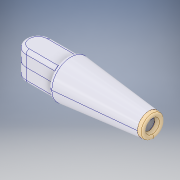
# Autodesk Inventor part: SimplifiedFoot040x
Saved by Autodesk Inventor 2018 (Build 220112000, 112)
## iProperties
Part Number: SimplifiedFoot040x
Material: PVC, hart
Document SubType Name: Modeling
Designer: Jochen Alt
Mass: 40.2314 g
Surface Area: 453.473 cm^2
Volume: 40.2314 cm^3
Density: 1.29 g/cm^3
Appearance: Glatt - waldgrün
Author: Jochen Alt
Autodesk Inventor part; units mm, degrees
(part 1 of 2)
ref_plane "YZ Plane" through (0, 0, 0) normal (1, 0, 0) x (0, 1, 0)
ref_plane "XZ Plane" through (0, 0, 0) normal (0, 1, 0) x (-1, 0, 0)
ref_plane "XY Plane" through (0, 0, 0) normal (0, 0, 1) x (1, 0, 0)
sketch "Skizze Servo Projektion" plane through (0, 0, 0) normal (0, 0, 1) x (1, 0, 0)
  circle A0 centre (6.3, 9) radius 0.85 construction
  circle A1 centre (6.3, -9) radius 0.85 construction
  circle A2 centre (-32.7, -9) radius 0.85 construction
  circle A3 centre (-32.7, 9) radius 0.85 construction
  circle A4 centre (-26.0282, 0) radius 9.5 construction
  line L0 (0.03, 10) -> (0.03, 11.5) construction
  arc A5 (0.03, 10) -> (1.9, 8.13) centre (1.9, 10) ccw construction
  line L1 (3.3264, 8.13) -> (1.9, 8.13) construction
  arc A6 (3.8197, 7.7121) -> (3.3264, 8.13) centre (3.3264, 7.63) ccw construction
  arc A7 (3.8197, 7.7121) -> (5.25, 6.5) centre (5.25, 7.95) ccw construction
  line L2 (5.25, 6.5) -> (9, 6.5) construction
  line L3 (9, 8.0017) -> (9, 6.5) construction
  arc A8 (9.0005, 8.0017) -> (5.3017, 11.7005) centre (5.3, 8) ccw construction
  line L4 (3.75, 11.7) -> (5.3017, 11.7) construction
  line L5 (3.75, 11.7) -> (3.75, 10.9) construction
  line L6 (3.75, 10.9) -> (3.4008, 10.9) construction
  arc A9 (1.15, 11.5811) -> (3.4008, 10.9) centre (1.9, 10) ccw construction
  line L7 (1.15, 11.7) -> (1.15, 11.5811) construction
  line L8 (-0.0117, 11.7) -> (1.15, 11.7) construction
  arc A10 (0.03, 11.5) -> (-0.0117, 11.7) centre (-0.47, 11.5) ccw construction
  arc A11 (6.3002, 10.3002) -> (6.3, 7.6998) centre (6.3, 9) ccw construction
  arc A12 (6.3, 7.6996) -> (6.3002, 10.3004) centre (6.3, 9) ccw construction
  line L9 (-0.0117, -11.7) -> (1.15, -11.7) construction
  line L10 (1.15, -11.7) -> (1.15, -11.5811) construction
  arc A13 (3.4008, -10.9) -> (1.15, -11.5811) centre (1.9, -10) ccw construction
  line L11 (3.75, -10.9) -> (3.4008, -10.9) construction
  line L12 (3.75, -11.7) -> (3.75, -10.9) construction
  line L13 (5.3017, -11.7) -> (3.75, -11.7) construction
  arc A14 (5.3017, -11.7005) -> (9.0005, -8.0017) centre (5.3, -8) ccw construction
  line L14 (9, -6.5) -> (9, -8.0017) construction
  line L15 (9, -6.5) -> (5.25, -6.5) construction
  arc A15 (5.25, -6.5) -> (3.8197, -7.7121) centre (5.25, -7.95) ccw construction
  arc A16 (3.3264, -8.13) -> (3.8197, -7.7121) centre (3.3264, -7.63) ccw construction
  line L16 (3.3264, -8.13) -> (1.9, -8.13) construction
  arc A17 (1.9, -8.13) -> (0.03, -10) centre (1.9, -10) ccw construction
  line L17 (0.03, -10) -> (0.03, -11.5) construction
  arc A18 (-0.0117, -11.7) -> (0.03, -11.5) centre (-0.47, -11.5) ccw construction
  arc A19 (6.2998, -7.6997) -> (6.3, -10.3003) centre (6.3, -9) ccw construction
  arc A20 (6.3, -10.3002) -> (6.2998, -7.6998) centre (6.3, -9) ccw construction
  line L18 (-34.4734, 6.5) -> (-34.4734, 6.702) construction
  line L19 (-30.9117, 6.702) -> (-34.4734, 6.702) construction
  arc A21 (-30.9117, 6.702) -> (-30.2197, 7.7121) centre (-31.65, 7.95) ccw construction
  arc A22 (-29.7264, 8.13) -> (-30.2197, 7.7121) centre (-29.7264, 7.63) ccw construction
  line L20 (-29.7264, 8.13) -> (-28.3, 8.13) construction
  arc A23 (-28.3, 8.13) -> (-26.43, 10) centre (-28.3, 10) ccw construction
  line L21 (-26.43, 11.7) -> (-26.43, 10) construction
  line L22 (-27.55, 11.7) -> (-26.43, 11.7) construction
  line L23 (-27.55, 11.7) -> (-27.55, 11.5811) construction
  arc A24 (-29.8008, 10.9) -> (-27.55, 11.5811) centre (-28.3, 10) ccw construction
  line L24 (-30.15, 10.9) -> (-29.8008, 10.9) construction
  line L25 (-30.15, 11.7) -> (-30.15, 10.9) construction
  line L26 (-31.7017, 11.7) -> (-30.15, 11.7) construction
  arc A25 (-31.7017, 11.7005) -> (-35.4005, 8.0017) centre (-31.7, 8) ccw construction
  line L27 (-35.4, 6.5) -> (-35.4, 8.0017) construction
  line L28 (-35.4, 6.5) -> (-34.4734, 6.5) construction
  circle A26 centre (-32.7, 9) radius 1.3004 construction
  line L29 (-30.4301, -7.1662) -> (-34.4734, -7.1662) construction
  line L30 (-34.4734, -6.5) -> (-34.4734, -7.1662) construction
  line L31 (-34.4734, -6.5) -> (-35.4, -6.5) construction
  line L32 (-35.4, -8.0012) -> (-35.4, -6.5) construction
  arc A27 (-35.4005, -8.0012) -> (-31.7017, -11.7005) centre (-31.7, -8) ccw construction
  line L33 (-30.15, -11.7) -> (-31.7017, -11.7) construction
  line L34 (-30.15, -11.7) -> (-30.15, -10.9) construction
  line L35 (-30.15, -10.9) -> (-29.8008, -10.9) construction
  arc A28 (-27.55, -11.5811) -> (-29.8008, -10.9) centre (-28.3, -10) ccw construction
  line L36 (-27.55, -11.7) -> (-27.55, -11.5811) construction
  line L37 (-26.43, -11.7) -> (-27.55, -11.7) construction
  line L38 (-26.43, -11.7) -> (-26.43, -10) construction
  arc A29 (-26.43, -10) -> (-28.3, -8.13) centre (-28.3, -10) ccw construction
  line L39 (-29.7264, -8.13) -> (-28.3, -8.13) construction
  arc A30 (-30.2197, -7.7121) -> (-29.7264, -8.13) centre (-29.7264, -7.63) ccw construction
  arc A31 (-30.2197, -7.7121) -> (-30.4301, -7.1662) centre (-31.65, -7.95) ccw construction
  circle A32 centre (-32.7, -9) radius 1.3004 construction
  line L40 (-35.4, 8.0001) -> (-35.4, 6.5) construction
  arc A33 (-31.7001, 11.7) -> (-35.4, 8.0001) centre (-31.7, 8) ccw construction
  line L41 (-30.2, 11.7) -> (-31.7001, 11.7) construction
  line L42 (-30.2, 7.95) -> (-30.2, 11.7) construction
  arc A34 (-31.65, 6.5) -> (-30.2, 7.95) centre (-31.65, 7.95) ccw construction
  line L43 (-35.4, 6.5) -> (-31.65, 6.5) construction
  circle A35 centre (-32.7, 9) radius 1 construction
  line L44 (-31.7001, -11.7) -> (-30.2, -11.7) construction
  arc A36 (-35.4, -8.0001) -> (-31.7001, -11.7) centre (-31.7, -8) ccw construction
  line L45 (-35.4, -6.5) -> (-35.4, -8.0001) construction
  line L46 (-35.4, -6.5) -> (-31.65, -6.5) construction
  arc A37 (-30.2, -7.95) -> (-31.65, -6.5) centre (-31.65, -7.95) ccw construction
  line L47 (-30.2, -7.95) -> (-30.2, -11.7) construction
  circle A38 centre (-32.7, -9) radius 1 construction
  line L48 (3.8, -11.4999) -> (3.8, -7.95) construction
  arc A39 (5.25, -6.5) -> (3.8, -7.95) centre (5.25, -7.95) ccw construction
  line L49 (5.25, -6.5) -> (8.9886, -6.5) construction
  ellipse E0 centre (8.9925, -6.4605) end of major axis (8.8053, -6.4614) minor radius 0.0394 (8.9886, -6.5) -> (9, -6.4999) ccw construction
  line L50 (9, -8) -> (9, -6.4999) construction
  arc A40 (5.3, -11.7) -> (9, -8) centre (5.3, -8) ccw construction
  line L51 (3.7582, -11.7) -> (5.3, -11.7) construction
  arc A41 (3.7582, -11.7) -> (3.8, -11.4999) centre (3.2999, -11.4999) ccw construction
  circle A42 centre (6.3, -9) radius 1 construction
  line L52 (3.7582, 11.7) -> (5.3, 11.7) construction
  arc A43 (9, 8) -> (5.3, 11.7) centre (5.3, 8) ccw construction
  line L53 (9, 6.4999) -> (9, 8) construction
  ellipse E1 centre (8.9925, 6.4605) end of major axis (8.8053, 6.4614) minor radius 0.0394 (9, 6.4999) -> (8.9886, 6.5) ccw construction
  line L54 (5.25, 6.5) -> (8.9886, 6.5) construction
  arc A44 (3.8, 7.95) -> (5.25, 6.5) centre (5.25, 7.95) ccw construction
  line L55 (3.8, 11.4999) -> (3.8, 7.95) construction
  arc A45 (3.8, 11.4999) -> (3.7582, 11.7) centre (3.2999, 11.4999) ccw construction
  circle A46 centre (6.3, 9) radius 1 construction
  line L56 (-14.1, 10.2) -> (-14.1, -10.2) construction
  line L57 (-9.1, -10.2) -> (-9.1, 10.2) construction
  line L58 (-3.4016, 1.5) -> (3.0621, 1.5) construction
  ellipse E2 centre (-3.3983, 1.8017) end of major axis (-3.6128, 1.5872) minor radius 0.3 (-3.7, 1.7984) -> (-3.4016, 1.5) ccw construction
  line L59 (-3.7, 2.5) -> (-3.7, 1.7984) construction
  line L60 (-8.6653, 4.1133) -> (-3.7, 2.5) construction
  ellipse E3 centre (-8.4844, 4.5832) end of major axis (-9.0452, 4.6462) minor radius 0.5 (-9.048, 4.5967) -> (-8.6653, 4.1133) ccw construction
  line L61 (-9.048, -4.5967) -> (-9.048, 4.5967) construction
  ellipse E4 centre (-8.4844, -4.5832) end of major axis (-9.0452, -4.6462) minor radius 0.5 (-8.6653, -4.1133) -> (-9.048, -4.5967) ccw construction
  line L62 (-3.7, -2.5) -> (-8.6653, -4.1133) construction
  line L63 (-3.7, -2.5) -> (-3.7, -1.7984) construction
  ellipse E5 centre (-3.3983, -1.8017) end of major axis (-3.6128, -1.5872) minor radius 0.3 (-3.4016, -1.5) -> (-3.7, -1.7984) ccw construction
  line L64 (-3.4016, -1.5) -> (3.0621, -1.5) construction
  ellipse E6 centre (3.0403, -3.5108) end of major axis (1.6076, -4.9373) minor radius 1.9999 (4.5504, -2.1667) -> (3.0621, -1.5) ccw construction
  ellipse E7 centre (5.3055, -1.4945) end of major axis (4.5906, -2.2094) minor radius 1 (4.5504, -2.1667) -> (5.2945, -2.5) ccw construction
  line L65 (9, -2.5) -> (5.2945, -2.5) construction
  line L66 (9, 2.5) -> (9, -2.5) construction
  line L67 (9, 2.5) -> (5.2945, 2.5) construction
  ellipse E8 centre (5.3055, 1.4945) end of major axis (4.5906, 2.2094) minor radius 1 (5.2945, 2.5) -> (4.5504, 2.1667) ccw construction
  ellipse E9 centre (3.0403, 3.5108) end of major axis (1.6077, 4.9373) minor radius 1.9999 (3.0621, 1.5) -> (4.5504, 2.1667) ccw construction
  circle A47 centre (0, 0) radius 1 construction
  line L68 (-7.0181, -1.8024) -> (-7.0181, -1.25) construction
  arc A48 (-7.0181, 1.7382) -> (-7.0181, -1.8024) centre (-7.1503, -0.0321) ccw construction
  line L69 (-7.0181, 1.1858) -> (-7.0181, 1.7382) construction
  arc A49 (-7.0181, 1.1858) -> (-7.0181, -1.25) centre (-7.1503, -0.0321) ccw construction
  line L70 (-4.4623, -0.3083) -> (-4.4623, 0.2441) construction
  line L71 (-5.409, -0.3083) -> (-4.4623, -0.3083) construction
  arc A50 (-5.409, -0.3083) -> (-4.0833, -1.25) centre (-4.2155, -0.0321) ccw construction
  line L72 (-4.0833, -1.8024) -> (-4.0833, -1.25) construction
  arc A51 (-4.0833, 1.7382) -> (-4.0833, -1.8024) centre (-4.2155, -0.0321) ccw construction
  line L73 (-4.0833, 1.1858) -> (-4.0833, 1.7382) construction
  arc A52 (-4.0833, 1.1858) -> (-5.409, 0.2441) centre (-4.2155, -0.0321) ccw construction
  line L74 (-4.4623, 0.2441) -> (-5.409, 0.2441) construction
  line L75 (-13.7722, 12) -> (-9.4278, 12) construction
  line L76 (-9.4278, -12) -> (-13.7722, -12) construction
  line L77 (9.3, 2.7701) -> (9.3, -2.7701) construction
  line L78 (-35.7, -6.2) -> (-35.7, 6.2) construction
  arc A53 (-31.7001, 12) -> (-35.7, 8.0001) centre (-31.7, 8) ccw construction
  arc A54 (9.3, 8.0001) -> (5.3001, 12) centre (5.3, 8) ccw construction
  arc A55 (5.3001, -12) -> (9.3, -8.0001) centre (5.3, -8) ccw construction
  arc A56 (-35.7, -8.0001) -> (-31.7001, -12) centre (-31.7, -8) ccw construction
  line L79 (-26.0282, 14.9066) -> (11.3, 14.9066)
  line L80 (11.3, 14.9066) -> (11.3, -14.9066)
  line L81 (11.3, -14.9066) -> (-26.0282, -14.9066)
  line L82 (18.4014, 0) -> (11.3, 0) construction
  line L83 (0, 0) -> (-45.3062, 0) construction
  arc A57 (-26.0282, 14.9066) -> (-26.0282, -14.9066) centre (-26.0282, 0) ccw
  line L84 (18.4014, 0) -> (-45.3062, 0) construction
  line L85 (18.4014, 0) -> (-45.3062, 0) construction
  line L86 (0, -17.8457) -> (0, 16.9839) construction
  line L87 (9.4, -8) -> (9.4, 8)
  line L88 (5.3, 12.1) -> (-31.7, 12.1)
  line L89 (-31.7, -12.1) -> (5.3, -12.1)
  line L90 (-35.8, -8) -> (-35.8, 8)
  arc A58 (-35.8, -8) -> (-31.7, -12.1) centre (-31.7, -8) ccw
  arc A59 (5.3, -12.1) -> (9.4, -8) centre (5.3, -8) ccw
  arc A60 (9.4, 8) -> (5.3, 12.1) centre (5.3, 8) ccw
  arc A61 (-31.7, 12.1) -> (-35.8, 8) centre (-31.7, 8) ccw
  line L91 (9.4, -6.6) -> (5.25, -6.6)
  line L92 (-31.65, -6.6) -> (-35.8, -6.6)
  line L93 (3.9, -12.1) -> (3.9, -7.95)
  line L94 (3.9, 7.95) -> (3.9, 12.1)
  line L95 (3.9, -1.6838) -> (3.9, -1.5)
  line L96 (3.9, -0.3083) -> (3.9, 0)
  line L97 (5.25, 6.6) -> (9.4, 6.6)
  line L98 (-35.8, 6.6) -> (-31.65, 6.6)
  line L99 (-34.0713, 11.3447) -> (-34.6497, 12.1605) construction
  arc A62 (5.25, -6.6) -> (3.9, -7.95) centre (5.25, -7.95) ccw
  arc A63 (3.9, 7.95) -> (5.25, 6.6) centre (5.25, 7.95) ccw
  line L100 (-30.3, -12.1) -> (-30.3, -7.95)
  line L101 (-30.3, 7.95) -> (-30.3, 12.1)
  arc A64 (-30.3, -7.95) -> (-31.65, -6.6) centre (-31.65, -7.95) ccw
  arc A65 (-31.65, 6.6) -> (-30.3, 7.95) centre (-31.65, 7.95) ccw
  line L102 (-14.1, -12.1) -> (-14.1, 12.1)
  line L103 (-9.1, -12.1) -> (-9.1, 12.1)
  arc A66 (-31.6484, 12.1) -> (-31.6491, 12.0997) centre (-26.0282, 0) ccw
  arc A67 (-35.5333, 9.4546) -> (-35.5333, -9.4546) centre (-26.0282, 0) ccw
  arc A68 (-31.6491, -12.0997) -> (-31.6484, -12.1) centre (-26.0282, 0) ccw
  circle A69 centre (-32.7, -9) radius 1.05
  circle A70 centre (-32.7, 9) radius 1.05
  circle A71 centre (6.3, 9) radius 1.05
  circle A72 centre (6.3, -9) radius 1.05
  dimension "d801" = 0.1
  dimension "d802" = 0.1
  dimension "d803" = 0.1
  dimension "d804" = 0.1
  dimension "d805" = 4.1
  dimension "d806" = 4.1
  dimension "d811" = 1
  dimension "d812" = 1.9
  dimension "d813" = 1.35
  dimension "d815" = 0.1
  dimension "d816" = 0.1
  dimension "d817" = 1.35
  dimension "d818" = 1.5
  dimension "d819" = 2.1
  dimension "d820" = 2.1
  dimension "d821" = 2.1
  dimension "d822" = 2.1
  constraints: 50 end point, 30 point on circle, 18 point on line, 18 tangent, 16 centre point, 9 horizontal, 7 vertical, 6 coincident, 5 parallel, 4 equal radius, 3 perpendicular, 2 collinear, 2 line through centre, 1 midpoint, 21 other
  measures "d801" distance between parallel lines of L77 L87
  measures "d802" distance between parallel lines of L75 L88
  measures "d803" distance between parallel lines of L76 L89
  measures "d804" distance between parallel lines of L90 L78
  measures "d805" radius of A58
  measures "d806" radius of A59
  measures "d811" distance of L99.end L99.start
  measures "d812" distance between parallel lines of L80 L87
  measures "d813" radius of A62
  measures "d815" distance between parallel lines of L55 L94
  measures "d816" distance between parallel lines of L100 L47
  measures "d817" radius of A64
  measures "d818" radial gap between concentric circles of A57 A67
  measures "d819" diameter of A69
  measures "d820" diameter of A70
  measures "d821" diameter of A71
  measures "d822" diameter of A72
extrude "Extrusion3" add sketch "Skizze Servo Projektion" against normal blind 35.2 contours L79 L80 L81 A57 | A59 L89 L93 A62 L91 L87 | L91 A62 L93 L89 L103 L88 L94 A63 L97 L87 | L97 A63 L94 L88 A60 L87 | L89 L102 A66 L88 L103 | L89 A66 L102 | A66 L89 | L89 L100 A64 L92 L90 L98 A65 L101 L88 A66 L102 | L102 A66 | L102 A66 L88 | L89 A66 A58 L90 L92 A64 L100 | L89 A58 A66 | L88 A66 | A66 A61 L90 A58 | A58 A67 A61 A66 | L101 A65 L98 L90 A61 A66 L88 | A66 A61 L88 | A69 | A70 | A71 | A72
ref_plane "Arbeitsebene23" through (9.8, -14.9066, 0) normal (1, 0, 0) x (0, 0, -1)
sketch "Skizze49" plane through (9.8, -14.9066, 0) normal (1, 0, 0) x (0, 0, -1)
  circle A0 centre (17.5, 15) radius 24
  point P0 (0, 14.9066)
  dimension "d270" = 48
  constraints: 1 centre point
  measures "d270" diameter of A0
extrude "Zylinder" add sketch "Skizze49" along normal blind 100 separate body
sketch "Skizze4" plane through (0, 0, 0) normal (0, 0, 1) x (1, 0, 0)
  circle A0 centre (-26.0282, 0) radius 5.8
  arc A1 (-26.0282, 14.9066) -> (-26.0282, -14.9066) centre (-26.0282, 0) ccw projected
  point P0 (0, 0)
  dimension "d16" = 11.6
  constraints: 1 centre point, 1 coincident
  measures "d16" diameter of A0
extrude "Extrusion4" [suppressed]
ref_plane "Arbeitsebene2" through (0, 0, -2.8) normal (0, 0, 1) x (1, 0, 0)
sketch "Skizze145" plane through (0, 0, -2.8) normal (0, 0, 1) x (1, 0, 0)
  line L0 (5.3, 12.1) -> (-31.7, 12.1) projected
  arc A0 (9.4, 8) -> (5.3, 12.1) centre (5.3, 8) ccw projected
  line L1 (9.4, -8) -> (9.4, 8) projected
  arc A1 (5.3, -12.1) -> (9.4, -8) centre (5.3, -8) ccw projected
  line L2 (-31.7, -12.1) -> (5.3, -12.1) projected
  arc A2 (-35.8, -8) -> (-31.7, -12.1) centre (-31.7, -8) ccw projected
  line L3 (-35.8, -8) -> (-35.8, 8) projected
  arc A3 (-31.7, 12.1) -> (-35.8, 8) centre (-31.7, 8) ccw projected
  line L4 (5.25, 6.6) -> (9.4, 6.6) projected
  arc A4 (3.9, 7.95) -> (5.25, 6.6) centre (5.25, 7.95) ccw projected
  circle A5 centre (6.3, 9) radius 1.05 projected
  line L5 (3.9, -12.1) -> (3.9, -7.95) projected
  line L6 (11.3, -14.9066) -> (11.3, 14.9066) projected
  line L7 (11.3, 14.9066) -> (-26.0282, 14.9066) projected
  arc A6 (-26.0282, 14.9066) -> (-26.0282, -14.9066) centre (-26.0282, 0) ccw projected
  line L8 (-26.0282, -14.9066) -> (11.3, -14.9066) projected
  circle A7 centre (6.3, -9) radius 1.05 projected
  arc A8 (5.25, -6.6) -> (3.9, -7.95) centre (5.25, -7.95) ccw projected
  line L9 (9.4, -6.6) -> (5.25, -6.6) projected
  line L10 (3.9, 7.95) -> (3.9, 12.1) projected
  point P0 (0, 0)
extrude "Extrusion105" [suppressed]
sketch "Skizze149" plane through (0, 0, -2.8) normal (0, 0, -1) x (-1, 0, 0)
  line L0 (35.8, -8) -> (35.8, 8) projected
  arc A0 (35.5333, -9.4546) -> (35.5333, 9.4546) centre (26.0282, 0) ccw projected
  arc A1 (31.7, -12.1) -> (35.8, -8) centre (31.7, -8) ccw projected
  arc A2 (35.8, 8) -> (31.7, 12.1) centre (31.7, 8) ccw projected
  point P0 (0, 0)
extrude "Extrusion108" [suppressed]
chamfer "Fase11" [suppressed]
chamfer "Fase14" [suppressed]
chamfer "Fase15" [suppressed]
extrude "Extrusion106" [suppressed]
ref_plane "Arbeitsebene3" through (0, 0, -34.4) normal (0, 0, 1) x (1, 0, 0)
sketch "Skizze146" plane through (0, 0, -34.4) normal (0, 0, 1) x (1, 0, 0)
  line L0 (3.9, -12.1) -> (3.9, -7.95) projected
  line L1 (-31.7, -12.1) -> (5.3, -12.1) projected
  arc A0 (5.3, -12.1) -> (9.4, -8) centre (5.3, -8) ccw projected
  line L2 (9.4, -8) -> (9.4, 8) projected
  line L3 (9.4, -6.6) -> (5.25, -6.6) projected
  arc A1 (5.25, -6.6) -> (3.9, -7.95) centre (5.25, -7.95) ccw projected
  circle A2 centre (6.3, -9) radius 1.05 projected
  line L4 (5.25, 6.6) -> (9.4, 6.6) projected
  arc A3 (3.9, 7.95) -> (5.25, 6.6) centre (5.25, 7.95) ccw projected
  line L5 (3.9, 7.95) -> (3.9, 12.1) projected
  arc A4 (9.4, 8) -> (5.3, 12.1) centre (5.3, 8) ccw projected
  circle A5 centre (6.3, 9) radius 1 construction
  circle A6 centre (6.3, 9) radius 1.05 projected
  line L6 (5.3, 12.1) -> (-31.7, 12.1) projected
  line L7 (-35.8, 6.6) -> (-31.65, 6.6) projected
  arc A7 (-31.65, 6.6) -> (-30.3, 7.95) centre (-31.65, 7.95) ccw projected
  line L8 (-30.3, 7.95) -> (-30.3, 12.1) projected
  arc A8 (-31.7, 12.1) -> (-35.8, 8) centre (-31.7, 8) ccw projected
  line L9 (-35.8, -8) -> (-35.8, 8) projected
  line L10 (-31.65, -6.6) -> (-35.8, -6.6) projected
  arc A9 (-30.3, -7.95) -> (-31.65, -6.6) centre (-31.65, -7.95) ccw projected
  line L11 (-30.3, -12.1) -> (-30.3, -7.95) projected
  arc A10 (-35.8, -8) -> (-31.7, -12.1) centre (-31.7, -8) ccw projected
  circle A11 centre (-32.7, -9) radius 1.05 projected
  circle A12 centre (-32.7, 9) radius 1.05 projected
  point P0 (0, 0)
extrude "Extrusion107" [suppressed]
sketch "Skizze5" plane through (0, 0, -35.2) normal (0, 0, -1) x (-1, 0, 0)
  arc A0 (26.0282, -14.9066) -> (26.0282, 14.9066) centre (26.0282, 0) ccw projected
  circle A1 centre (26.0282, 0) radius 9.75
  point P0 (0, 0)
  dimension "d19" = 19.5
  constraints: 1 centre point, 1 coincident
  measures "d19" diameter of A1
extrude "Extrusion5" [suppressed]
ref_plane "Arbeitsebene6" through (0, 0, 0) normal (0, 0, 1) x (1, 0, 0)
sketch "Skizze11" plane through (0, 0, 0) normal (0, 0, 1) x (1, 0, 0)
  circle A0 centre (6.3, 9) radius 0.85 construction
  circle A1 centre (6.3, -9) radius 0.85 construction
  circle A2 centre (-32.7, -9) radius 0.85 construction
  circle A3 centre (-32.7, 9) radius 0.85 construction
  circle A4 centre (-26.0282, 0) radius 9.5 construction
  line L0 (0.03, 10) -> (0.03, 11.5) construction
  arc A5 (0.03, 10) -> (1.9, 8.13) centre (1.9, 10) ccw construction
  line L1 (3.3264, 8.13) -> (1.9, 8.13) construction
  arc A6 (3.8197, 7.7121) -> (3.3264, 8.13) centre (3.3264, 7.63) ccw construction
  arc A7 (3.8197, 7.7121) -> (5.25, 6.5) centre (5.25, 7.95) ccw construction
  line L2 (5.25, 6.5) -> (9, 6.5) construction
  line L3 (9, 8.0017) -> (9, 6.5) construction
  arc A8 (9.0005, 8.0017) -> (5.3017, 11.7005) centre (5.3, 8) ccw construction
  line L4 (3.75, 11.7) -> (5.3017, 11.7) construction
  line L5 (3.75, 11.7) -> (3.75, 10.9) construction
  line L6 (3.75, 10.9) -> (3.4008, 10.9) construction
  arc A9 (1.15, 11.5811) -> (3.4008, 10.9) centre (1.9, 10) ccw construction
  line L7 (1.15, 11.7) -> (1.15, 11.5811) construction
  line L8 (-0.0117, 11.7) -> (1.15, 11.7) construction
  arc A10 (0.03, 11.5) -> (-0.0117, 11.7) centre (-0.47, 11.5) ccw construction
  arc A11 (6.3002, 10.3002) -> (6.3, 7.6998) centre (6.3, 9) ccw construction
  arc A12 (6.3, 7.6996) -> (6.3002, 10.3004) centre (6.3, 9) ccw construction
  line L9 (-0.0117, -11.7) -> (1.15, -11.7) construction
  line L10 (1.15, -11.7) -> (1.15, -11.5811) construction
  arc A13 (3.4008, -10.9) -> (1.15, -11.5811) centre (1.9, -10) ccw construction
  line L11 (3.75, -10.9) -> (3.4008, -10.9) construction
  line L12 (3.75, -11.7) -> (3.75, -10.9) construction
  line L13 (5.3017, -11.7) -> (3.75, -11.7) construction
  arc A14 (5.3017, -11.7005) -> (9.0005, -8.0017) centre (5.3, -8) ccw construction
  line L14 (9, -6.5) -> (9, -8.0017) construction
  line L15 (9, -6.5) -> (5.25, -6.5) construction
  arc A15 (5.25, -6.5) -> (3.8197, -7.7121) centre (5.25, -7.95) ccw construction
  arc A16 (3.3264, -8.13) -> (3.8197, -7.7121) centre (3.3264, -7.63) ccw construction
  line L16 (3.3264, -8.13) -> (1.9, -8.13) construction
  arc A17 (1.9, -8.13) -> (0.03, -10) centre (1.9, -10) ccw construction
  line L17 (0.03, -10) -> (0.03, -11.5) construction
  arc A18 (-0.0117, -11.7) -> (0.03, -11.5) centre (-0.47, -11.5) ccw construction
  arc A19 (6.2998, -7.6997) -> (6.3, -10.3003) centre (6.3, -9) ccw construction
  arc A20 (6.3, -10.3002) -> (6.2998, -7.6998) centre (6.3, -9) ccw construction
  line L18 (-34.4734, 6.5) -> (-34.4734, 6.702) construction
  line L19 (-30.9117, 6.702) -> (-34.4734, 6.702) construction
  arc A21 (-30.9117, 6.702) -> (-30.2197, 7.7121) centre (-31.65, 7.95) ccw construction
  arc A22 (-29.7264, 8.13) -> (-30.2197, 7.7121) centre (-29.7264, 7.63) ccw construction
  line L20 (-29.7264, 8.13) -> (-28.3, 8.13) construction
  arc A23 (-28.3, 8.13) -> (-26.43, 10) centre (-28.3, 10) ccw construction
  line L21 (-26.43, 11.7) -> (-26.43, 10) construction
  line L22 (-27.55, 11.7) -> (-26.43, 11.7) construction
  line L23 (-27.55, 11.7) -> (-27.55, 11.5811) construction
  arc A24 (-29.8008, 10.9) -> (-27.55, 11.5811) centre (-28.3, 10) ccw construction
  line L24 (-30.15, 10.9) -> (-29.8008, 10.9) construction
  line L25 (-30.15, 11.7) -> (-30.15, 10.9) construction
  line L26 (-31.7017, 11.7) -> (-30.15, 11.7) construction
  arc A25 (-31.7017, 11.7005) -> (-35.4005, 8.0017) centre (-31.7, 8) ccw construction
  line L27 (-35.4, 6.5) -> (-35.4, 8.0017) construction
  line L28 (-35.4, 6.5) -> (-34.4734, 6.5) construction
  circle A26 centre (-32.7, 9) radius 1.3004 construction
  line L29 (-30.4301, -7.1662) -> (-34.4734, -7.1662) construction
  line L30 (-34.4734, -6.5) -> (-34.4734, -7.1662) construction
  line L31 (-34.4734, -6.5) -> (-35.4, -6.5) construction
  line L32 (-35.4, -8.0012) -> (-35.4, -6.5) construction
  arc A27 (-35.4005, -8.0012) -> (-31.7017, -11.7005) centre (-31.7, -8) ccw construction
  line L33 (-30.15, -11.7) -> (-31.7017, -11.7) construction
  line L34 (-30.15, -11.7) -> (-30.15, -10.9) construction
  line L35 (-30.15, -10.9) -> (-29.8008, -10.9) construction
  arc A28 (-27.55, -11.5811) -> (-29.8008, -10.9) centre (-28.3, -10) ccw construction
  line L36 (-27.55, -11.7) -> (-27.55, -11.5811) construction
  line L37 (-26.43, -11.7) -> (-27.55, -11.7) construction
  line L38 (-26.43, -11.7) -> (-26.43, -10) construction
  arc A29 (-26.43, -10) -> (-28.3, -8.13) centre (-28.3, -10) ccw construction
  line L39 (-29.7264, -8.13) -> (-28.3, -8.13) construction
  arc A30 (-30.2197, -7.7121) -> (-29.7264, -8.13) centre (-29.7264, -7.63) ccw construction
  arc A31 (-30.2197, -7.7121) -> (-30.4301, -7.1662) centre (-31.65, -7.95) ccw construction
  circle A32 centre (-32.7, -9) radius 1.3004 construction
  line L40 (-35.4, 8.0001) -> (-35.4, 6.5) construction
  arc A33 (-31.7001, 11.7) -> (-35.4, 8.0001) centre (-31.7, 8) ccw construction
  line L41 (-30.2, 11.7) -> (-31.7001, 11.7) construction
  line L42 (-30.2, 7.95) -> (-30.2, 11.7) construction
  arc A34 (-31.65, 6.5) -> (-30.2, 7.95) centre (-31.65, 7.95) ccw construction
  line L43 (-35.4, 6.5) -> (-31.65, 6.5) construction
  circle A35 centre (-32.7, 9) radius 1 construction
  line L44 (-31.7001, -11.7) -> (-30.2, -11.7) construction
  arc A36 (-35.4, -8.0001) -> (-31.7001, -11.7) centre (-31.7, -8) ccw construction
  line L45 (-35.4, -6.5) -> (-35.4, -8.0001) construction
  line L46 (-35.4, -6.5) -> (-31.65, -6.5) construction
  arc A37 (-30.2, -7.95) -> (-31.65, -6.5) centre (-31.65, -7.95) ccw construction
  line L47 (-30.2, -7.95) -> (-30.2, -11.7) construction
  circle A38 centre (-32.7, -9) radius 1 construction
  line L48 (3.8, -11.4999) -> (3.8, -7.95) construction
  arc A39 (5.25, -6.5) -> (3.8, -7.95) centre (5.25, -7.95) ccw construction
  line L49 (5.25, -6.5) -> (8.9886, -6.5) construction
  ellipse E0 centre (8.9925, -6.4605) end of major axis (8.8053, -6.4614) minor radius 0.0394 (8.9886, -6.5) -> (9, -6.4999) ccw construction
  line L50 (9, -8) -> (9, -6.4999) construction
  arc A40 (5.3, -11.7) -> (9, -8) centre (5.3, -8) ccw construction
  line L51 (3.7582, -11.7) -> (5.3, -11.7) construction
  arc A41 (3.7582, -11.7) -> (3.8, -11.4999) centre (3.2999, -11.4999) ccw construction
  circle A42 centre (6.3, -9) radius 1 construction
  line L52 (3.7582, 11.7) -> (5.3, 11.7) construction
  arc A43 (9, 8) -> (5.3, 11.7) centre (5.3, 8) ccw construction
  line L53 (9, 6.4999) -> (9, 8) construction
  ellipse E1 centre (8.9925, 6.4605) end of major axis (8.8053, 6.4614) minor radius 0.0394 (9, 6.4999) -> (8.9886, 6.5) ccw construction
  line L54 (5.25, 6.5) -> (8.9886, 6.5) construction
  arc A44 (3.8, 7.95) -> (5.25, 6.5) centre (5.25, 7.95) ccw construction
  line L55 (3.8, 11.4999) -> (3.8, 7.95) construction
  arc A45 (3.8, 11.4999) -> (3.7582, 11.7) centre (3.2999, 11.4999) ccw construction
  circle A46 centre (6.3, 9) radius 1 construction
  line L56 (-14.1, 10.2) -> (-14.1, -10.2) construction
  line L57 (-9.1, -10.2) -> (-9.1, 10.2) construction
  line L58 (-3.4016, 1.5) -> (3.0621, 1.5) construction
  ellipse E2 centre (-3.3983, 1.8017) end of major axis (-3.6128, 1.5872) minor radius 0.3 (-3.7, 1.7984) -> (-3.4016, 1.5) ccw construction
  line L59 (-3.7, 2.5) -> (-3.7, 1.7984) construction
  line L60 (-8.6653, 4.1133) -> (-3.7, 2.5) construction
  ellipse E3 centre (-8.4844, 4.5832) end of major axis (-9.0452, 4.6462) minor radius 0.5 (-9.048, 4.5967) -> (-8.6653, 4.1133) ccw construction
  line L61 (-9.048, -4.5967) -> (-9.048, 4.5967) construction
  ellipse E4 centre (-8.4844, -4.5832) end of major axis (-9.0452, -4.6462) minor radius 0.5 (-8.6653, -4.1133) -> (-9.048, -4.5967) ccw construction
  line L62 (-3.7, -2.5) -> (-8.6653, -4.1133) construction
  line L63 (-3.7, -2.5) -> (-3.7, -1.7984) construction
  ellipse E5 centre (-3.3983, -1.8017) end of major axis (-3.6128, -1.5872) minor radius 0.3 (-3.4016, -1.5) -> (-3.7, -1.7984) ccw construction
  line L64 (-3.4016, -1.5) -> (3.0621, -1.5) construction
  ellipse E6 centre (3.0403, -3.5108) end of major axis (1.6076, -4.9373) minor radius 1.9999 (4.5504, -2.1667) -> (3.0621, -1.5) ccw construction
  ellipse E7 centre (5.3055, -1.4945) end of major axis (4.5906, -2.2094) minor radius 1 (4.5504, -2.1667) -> (5.2945, -2.5) ccw construction
  line L65 (9, -2.5) -> (5.2945, -2.5) construction
  line L66 (9, 2.5) -> (9, -2.5) construction
  line L67 (9, 2.5) -> (5.2945, 2.5) construction
  ellipse E8 centre (5.3055, 1.4945) end of major axis (4.5906, 2.2094) minor radius 1 (5.2945, 2.5) -> (4.5504, 2.1667) ccw construction
  ellipse E9 centre (3.0403, 3.5108) end of major axis (1.6077, 4.9373) minor radius 1.9999 (3.0621, 1.5) -> (4.5504, 2.1667) ccw construction
  circle A47 centre (0, 0) radius 1 construction
  line L68 (-7.0181, -1.8024) -> (-7.0181, -1.25) construction
  arc A48 (-7.0181, 1.7382) -> (-7.0181, -1.8024) centre (-7.1503, -0.0321) ccw construction
  line L69 (-7.0181, 1.1858) -> (-7.0181, 1.7382) construction
  arc A49 (-7.0181, 1.1858) -> (-7.0181, -1.25) centre (-7.1503, -0.0321) ccw construction
  line L70 (-4.4623, -0.3083) -> (-4.4623, 0.2441) construction
  line L71 (-5.409, -0.3083) -> (-4.4623, -0.3083) construction
  arc A50 (-5.409, -0.3083) -> (-4.0833, -1.25) centre (-4.2155, -0.0321) ccw construction
  line L72 (-4.0833, -1.8024) -> (-4.0833, -1.25) construction
  arc A51 (-4.0833, 1.7382) -> (-4.0833, -1.8024) centre (-4.2155, -0.0321) ccw construction
  line L73 (-4.0833, 1.1858) -> (-4.0833, 1.7382) construction
  arc A52 (-4.0833, 1.1858) -> (-5.409, 0.2441) centre (-4.2155, -0.0321) ccw construction
  line L74 (-4.4623, 0.2441) -> (-5.409, 0.2441) construction
  line L75 (-13.7722, 12) -> (-9.4278, 12) construction
  line L76 (-9.4278, -12) -> (-13.7722, -12) construction
  line L77 (9.3, 2.7701) -> (9.3, -2.7701) construction
  line L78 (-35.7, -6.2) -> (-35.7, 6.2) construction
  arc A53 (-31.7001, 12) -> (-35.7, 8.0001) centre (-31.7, 8) ccw construction
  arc A54 (9.3, 8.0001) -> (5.3001, 12) centre (5.3, 8) ccw construction
  arc A55 (5.3001, -12) -> (9.3, -8.0001) centre (5.3, -8) ccw construction
  arc A56 (-35.7, -8.0001) -> (-31.7001, -12) centre (-31.7, -8) ccw construction
  line L79 (-26.0282, 15) -> (11.3, 15)
  line L80 (11.3, 15) -> (11.3, -15)
  line L81 (11.3, -15) -> (-26.0282, -15)
  line L82 (18.4014, 0) -> (11.3, 0) construction
  line L83 (0, 0) -> (-45.3062, 0) construction
  arc A57 (-26.0282, 15) -> (-26.0282, -15) centre (-26.0282, 0) ccw
  line L84 (18.4014, 0) -> (-45.3062, 0) construction
  line L85 (18.4014, 0) -> (-45.3062, 0) construction
  line L86 (0, -17.8457) -> (0, 16.9839) construction
  dimension "d59" = 2
  dimension "d60" = 15
  constraints: 16 end point, 5 horizontal, 2 point on circle, 2 tangent, 1 centre point, 1 coincident, 1 midpoint, 1 parallel, 1 perpendicular, 1 vertical, 18 other
  measures "d59" distance between parallel lines of L80 L77
  measures "d60" radius of A57
sketch "Skizze12" plane through (0, 0, -35.2) normal (0, 0, -1) x (-1, 0, 0)
  circle A0 centre (-6.3, -9) radius 1.05 construction
  circle A1 centre (-6.3, 9) radius 1.05 construction
  point P0 (0, 0)
hole "Bohrung2" [suppressed]
sketch "Skizze147" plane through (0, 0, 0) normal (0, 0, 1) x (1, 0, 0)
  point P0 (0, 0)
  point P1 (6.3, -9)
  point P2 (6.3, -9)
  point P3 (6.3, 9.0312)
  constraints: 1 coincident
hole "Bohrung14" [suppressed]
ref_plane "Arbeitsebene Teilung" through (0, 0, -17.5) normal (0, 0, 1) x (1, 0, 0)
sketch "Skizze16" plane through (0, 0, -17.5) normal (0, 0, 1) x (1, 0, 0)
  circle A0 centre (-26.0282, 0) radius 5.8 construction
  arc A1 (-26.0282, 14.9066) -> (-26.0282, -14.9066) centre (-26.0282, 0) ccw construction
  line L0 (-26.0282, -14.9066) -> (11.3, -14.9066) construction
  line L1 (11.3, 14.9066) -> (-26.0282, 14.9066) construction
  line L2 (-78.3938, 0) -> (148.1656, 0) construction
  line L3 (0, -33.5066) -> (0, 33.6934) construction
  line L4 (-26.0282, 0) -> (-39.6681, -14.6271)
  line L5 (-26.0282, 0) -> (0.6303, 0) construction
  line L6 (-39.6681, -14.6271) -> (-26.0282, 0)
  line L7 (-26.0282, 0) -> (-39.6681, 14.6271)
  line L8 (-26.0282, 0) -> (2.3641, 0) construction
  circle A2 centre (-26.0282, 0) radius 5.8 projected
  arc A3 (-39.6681, 14.6271) -> (-39.6681, -14.6271) centre (-26.0282, 0) ccw
  point P0 (0, 0)
  point P1 (-0.7, -15)
  point P2 (-0.7, 15)
  point P3 (11.3, -14.9066)
  point P4 (9.8, -15)
  point P5 (9.8, 15)
  dimension "d80" = 133
  dimension "d81" = 133
  dimension "d82" = 40
  constraints: 10 end point, 2 horizontal, 2 point on circle, 1 centre point, 1 coincident, 1 collinear, 2 other
  measures "d80" angle of L4 L5
  measures "d81" angle of L8 L7
  measures "d82" diameter of A3
extrude "Extrusion11" cut sketch "Skizze16" along normal mid plane 4 contours L4 A2 L7 | L4 A3 L7 A2 picked at (-28.9576, 2.483) bodies 1
chamfer "Kegelfase" distance 10 distance2 100 1 edges at (109.8, 0.0934, 6.5) measured on face at (109.8, 0.0934, 6)
fillet "Rundung41" radius 4 2 edges at (9.8001, 0.0934, 6.5) (9.8, 0.0934, 6.5)
fillet "Rundung22" radius 2 4 edges at (-31.1113, -5.451, -15.5) (-31.1113, -5.451, -19.5) (-31.1113, 5.451, -15.5) (-31.1113, 5.451, -19.5)
fillet "Rundung27" radius 1 8 edges at (-36.1945, -10.902, -17.5) (-36.5482, -10.5611, -16.1871) (-36.5482, -10.5611, -18.8129) (-40.9348, 0, -19.5) (-36.5482, 10.5611, -18.8129) (-36.1945, 10.902, -17.5) (-36.5469, 10.5623, -16.1891) (-40.9348, 0, -15.5)
sketch "Skizze148" plane through (0, 0, -2.8) normal (0, 0, -1) x (-1, 0, 0)
  point P0 (0, 0)
sketch "Skizze72" plane through (109.8, 0.0934, -17.5) normal (1, 0, 0) x (0, 0, -1)
  circle A0 centre (0, 0) radius 14 projected
  circle A1 centre (0, 0) radius 10.5
  point P0 (-17.5, -0.0934)
  dimension "d456" = 21
  constraints: 1 centre point, 1 coincident
  measures "d456" diameter of A1
extrude "Dämpferloch" cut sketch "Skizze72" against normal blind 5.5 contours A1 bodies 2
fillet "Rundung2" radius 4 6 edges at (-40.9348, 0, -35.2) (-7.3641, -14.9066, -35.2) (-7.3641, 14.9066, -35.2) (-40.9348, 0, 0) (-7.3641, -14.9066, 0) (-7.3641, 14.9066, 0)
ref_plane "Ebene Hälftenschnitt" through (0, 0, -17.6) normal (0, 0, -1) x (-1, 0, 0)
sketch "Skizze73" plane through (0, 0, -17.6) normal (0, 0, -1) x (-1, 0, 0)
  circle A0 centre (-71.8, 0) radius 2.2 construction
  line L0 (-70.5298, 2.2) -> (-69.2597, 0)
  line L1 (-69.2597, 0) -> (-70.5298, -2.2)
  line L2 (-70.5298, -2.2) -> (-73.0702, -2.2)
  line L3 (-73.0702, -2.2) -> (-74.3403, 0)
  line L4 (-74.3403, 0) -> (-73.0702, 2.2)
  line L5 (-73.0702, 2.2) -> (-70.5298, 2.2)
  circle A1 centre (-71.8, 0) radius 1.05
  line L6 (-9.8, 20.0934) -> (-9.8, -19.9066) projected
  point P0 (0, 0)
  point P1 (-71.8, 2.2)
  dimension "d488" = 4.4
  dimension "d489" = 2.1
  dimension "d854" = 62
  constraints: 12 end point, 3 coincident, 1 centre point, 1 midpoint, 1 vertical alignment, 15 other
  measures "d489" diameter of A1
  measures "d854" distance from line of point (-71.8, 0) L6
extrude "Häfftentrenner Bolzen" [suppressed]
extrude "Häftentrenner Loch" [suppressed]
sketch "Skizze74" plane through (71.8, 0, 2.4) normal (0, 0, 1) x (1, 0, 0)
  circle A0 centre (0, 0) radius 1.05 projected
  circle A1 centre (0, 0) radius 2
  point P0 (-71.8, 0)
  dimension "d494" = 4
  constraints: 1 centre point, 1 coincident
  measures "d494" diameter of A1
extrude "Hälftentrenner Schraubkopf 1" [suppressed]
sketch "Skizze75" plane through (71.8, 0, -37.6) normal (0, 0, -1) x (-1, 0, 0)
  circle A0 centre (0, 0) radius 1.05 projected
  circle A1 centre (0, 0) radius 2
  point P0 (71.8, 0)
  dimension "d497" = 4
  constraints: 1 centre point, 1 coincident
  measures "d497" diameter of A1
extrude "Hälftentrenner Schraubkopf 2" [suppressed]
feature "Kombinieren5" [suppressed]
shell "Wandung7" thickness 1.5 removed faces 0 bodies 2
combine bodies "Kombinieren6" operation type add bodies to combine 1 2
sketch "Skizze151" plane through (0, 0, -2.8) normal (0, 0, -1) x (-1, 0, 0)
  line L0 (-3.9, 11.1) -> (-3.9, 7.95) projected
  arc A0 (-5.25, 6.6) -> (-3.9, 7.95) centre (-5.25, 7.95) ccw projected
  line L1 (-5.25, 6.6) -> (-8.4, 6.6) projected
  line L2 (-8.4, -6.6) -> (-8.4, 6.6) projected
  line L3 (-8.4, -6.6) -> (-5.25, -6.6) projected
  arc A1 (-3.9, -7.95) -> (-5.25, -6.6) centre (-5.25, -7.95) ccw projected
  line L4 (-3.9, -7.95) -> (-3.9, -11.1) projected
  line L5 (31.7, -11.1) -> (-3.9, -11.1) projected
  arc A2 (31.7, -11.1) -> (34.6642, -8.9075) centre (31.7, -8) ccw projected
  arc A3 (34.6642, -8.9075) -> (34.6642, 8.9075) centre (26.0282, 0) ccw projected
  arc A4 (34.6642, 8.9075) -> (31.7, 11.1) centre (31.7, 8) ccw projected
  line L6 (-3.9, 11.1) -> (31.7, 11.1) projected
  circle A5 centre (26.0282, 0) radius 5.8 projected
  circle A6 centre (26.0282, 0) radius 6.6
  line L7 (8.0282, -3) -> (-13.2377, -3)
  line L8 (8.0282, 3) -> (-13.2377, 3)
  line L9 (-18.4014, 0) -> (45.3062, 0) construction
  line L10 (-13.2377, -3) -> (-13.2377, 3)
  line L11 (8.0282, -11.1) -> (8.0282, -3)
  line L12 (8.0282, 3) -> (8.0282, 11.1)
  point P0 (0, 0)
  dimension "d869" = 0.8
  dimension "d872" = 6
  constraints: 10 end point, 2 horizontal, 2 parallel, 2 point on line, 1 centre point, 1 coincident, 1 vertical, 1 other
  measures "d869" radial gap between concentric circles of A6 A5
  measures "d872" distance between parallel lines of L8 L7
extrude "Extrusion112" [suppressed]
sketch "Skizze152" plane through (0, 0, -1) normal (0, 0, -1) x (-1, 0, 0)
  line L0 (-8.4, -3) -> (-8.4, 3) projected
  line L1 (-11.3, -3) -> (-8.4, -3) projected
  line L2 (-11.3, 3) -> (-11.3, -3) projected
  line L3 (-8.4, 3) -> (-11.3, 3) projected
  point P0 (0, 0)
extrude "Extrusion113" [suppressed]
sketch "Skizze150" plane through (0, 0, -2.8) normal (0, 0, -1) x (-1, 0, 0)
  circle A0 centre (26.0282, 0) radius 5.8 projected
  circle A1 centre (26.0282, 0) radius 6.6
  line L0 (0, 0) -> (45.3062, 0) construction
  line L1 (-11.3, -3) -> (-11.3, 3)
  line L2 (-11.3, 19.6734) -> (-11.3, -19.4867) projected
  line L3 (8.0282, -3) -> (-11.3, -3)
  line L4 (8.0282, 3) -> (-11.3, 3)
  line L5 (8.0282, -12.1) -> (8.0282, -3)
  line L6 (8.0282, 3) -> (8.0282, 12.1)
  line L7 (35.7, -6.2) -> (35.7, 6.2) construction
  line L8 (35.8, -8) -> (35.8, 8) projected
  arc A2 (35.8, 8) -> (31.7, 12.1) centre (31.7, 8) ccw projected
  arc A3 (35.5333, -9.4546) -> (35.5333, 9.4546) centre (26.0282, 0) ccw projected
  arc A4 (31.7, -12.1) -> (35.8, -8) centre (31.7, -8) ccw projected
  line L9 (31.7, -12.1) -> (-5.3, -12.1) projected
  line L10 (-5.3, 12.1) -> (31.7, 12.1) projected
  arc A5 (-5.3, 12.1) -> (-9.4, 8) centre (-5.3, 8) ccw projected
  line L11 (-9.4, -8) -> (-9.4, 8) projected
  arc A6 (-9.4, -8) -> (-5.3, -12.1) centre (-5.3, -8) ccw projected
  line L12 (8.0282, -3) -> (8.0282, 3)
  arc A7 (35.5333, 9.4546) -> (31.7, 12.1) centre (31.7, 8) ccw projected
  arc A8 (35.5333, -9.4546) -> (35.5333, 9.4546) centre (26.0282, 0) ccw projected
  line L13 (31.7, 12.1) -> (-3.9, 12.1) projected
  arc A9 (31.7, -12.1) -> (35.5333, -9.4546) centre (31.7, -8) ccw projected
  line L14 (-3.9, -12.1) -> (31.7, -12.1) projected
  line L15 (30.3, 11.1) -> (-3.9, 11.1) projected
  arc A10 (35.5333, 9.4546) -> (31.7, 12.1) centre (31.7, 8) ccw projected
  line L16 (31.7, 11.1) -> (31.7, 12.1) projected
  line L17 (-3.9, 12.1) -> (-3.9, 11.1) projected
  line L18 (-3.9, 11.1) -> (8.0282, 11.1) projected
  line L19 (31.7, 11.1) -> (31.7, 12.1) projected
  line L20 (31.7, 12.1) -> (-3.9, 12.1) projected
  arc A11 (35.5333, -9.4546) -> (35.5333, 9.4546) centre (26.0282, 0) ccw projected
  line L21 (31.7, -11.1) -> (31.7, -12.1) projected
  arc A12 (31.7, -12.1) -> (35.5333, -9.4546) centre (31.7, -8) ccw projected
  line L22 (-3.9, -11.1) -> (-3.9, -12.1) projected
  line L23 (-3.9, -12.1) -> (31.7, -12.1) projected
  line L24 (31.7, -11.1) -> (31.7, -12.1) projected
  line L25 (8.0282, -11.1) -> (-3.9, -11.1) projected
  circle A13 centre (-6.3, -9) radius 1.05 projected
  line L26 (-9.4, -8) -> (-9.4, -6.6) projected
  arc A14 (-9.4, -8) -> (-5.3, -12.1) centre (-5.3, -8) ccw projected
  line L27 (-3.9, -12.1) -> (-5.3, -12.1) projected
  line L28 (-3.9, -12.1) -> (-3.9, -7.95) projected
  arc A15 (-3.9, -7.95) -> (-5.25, -6.6) centre (-5.25, -7.95) ccw projected
  line L29 (-5.25, -6.6) -> (-9.4, -6.6) projected
  circle A16 centre (-6.3, 9.0312) radius 1.05 projected
  line L30 (-5.3, 12.1) -> (-3.9, 12.1) projected
  arc A17 (-5.3, 12.1) -> (-9.4, 8) centre (-5.3, 8) ccw projected
  line L31 (-9.4, 6.6) -> (-9.4, 8) projected
  line L32 (-9.4, 6.6) -> (-5.25, 6.6) projected
  arc A18 (-5.25, 6.6) -> (-3.9, 7.95) centre (-5.25, 7.95) ccw projected
  line L33 (-3.9, 7.95) -> (-3.9, 12.1) projected
  line L34 (-8.4, 6.6) -> (-9.4, 6.6) projected
  line L35 (-9.4, 6.6) -> (-9.4, 3) projected
  line L36 (-9.4, -6.6) -> (-8.4, -6.6) projected
  line L37 (-8.4, -6.6) -> (-8.4, -3) projected
  line L38 (-9.4, -3) -> (-9.4, -6.6) projected
  line L39 (-8.4, 3) -> (-8.4, 6.6) projected
  line L40 (31.7, -11.1) -> (8.0282, -11.1) projected
  arc A19 (31.7, -11.1) -> (34.6642, -8.9075) centre (31.7, -8) ccw projected
  arc A20 (34.6642, -8.9075) -> (34.6642, 8.9075) centre (26.0282, 0) ccw projected
  line L41 (8.0282, 11.1) -> (31.7, 11.1) projected
  arc A21 (34.6642, 8.9075) -> (31.7, 11.1) centre (31.7, 8) ccw projected
  line L42 (-8.4, -3) -> (-9.4, -3) projected
  line L43 (-9.4, 3) -> (-8.4, 3) projected
  dimension "d847" = 0.8
  dimension "d864" = 6
  dimension "d866" = 18
  constraints: 12 end point, 4 point on line, 3 vertical, 2 collinear, 2 horizontal, 1 centre point, 1 coincident, 5 other
  measures "d847" radial gap between concentric circles of A1 A0
  measures "d864" distance between parallel lines of L4 L3
  measures "d866" distance from line of L6 A0.centre
fillet "Rundung42" [suppressed]
fillet "Rundung38" radius 0.5 4 edges at (9.8, 0.0934, 0) (9.8, 14.9066, -17.5) (9.8, 0.0934, -35.2) (9.8, -14.9066, -17.5)
sketch "Skizze77" plane through (102.8, 0.0934, -17.5) normal (-1, 0, 0) x (0, 0, 1)
  line L0 (5, -7.8434) -> (-10.24, -7.8434) construction
  line L1 (-10.24, -7.8434) -> (-10.24, 7.6566) construction
  line L2 (-10.24, 7.6566) -> (5, 7.6566) construction
  line L3 (5, 7.6566) -> (5, -7.8434) construction
  line L4 (5, -7.8434) -> (-10.24, 7.6566) construction
  line L5 (-10.24, -7.8434) -> (5, 7.6566) construction
  line L6 (-33.0121, -0.0934) -> (33.0121, -0.0934) construction
  line L7 (-33.0121, -0.0934) -> (33.0121, -0.0934) construction
  line L8 (0, 33.0121) -> (0, -33.0121) construction
  circle A0 centre (5, -7.8434) radius 1.05
  circle A1 centre (5, 7.6566) radius 1.05
  circle A2 centre (5, -7.8434) radius 2
  circle A3 centre (5, 7.6566) radius 2
  circle A4 centre (0, 0) radius 10
  circle A5 centre (0, 0) radius 8
  point P0 (17.5, -0.0934)
  point P1 (-2.62, -0.0934)
  dimension "d509" = 15.24
  dimension "d510" = 15.5
  dimension "d512" = 5
  dimension "d513" = 2.1
  dimension "d514" = 2.1
  dimension "d515" = 4
  dimension "d516" = 4
  dimension "d527" = 20
  dimension "d532" = 16
  constraints: 12 end point, 6 centre point, 6 coincident, 2 midpoint, 2 parallel, 1 horizontal, 1 perpendicular, 1 point on line
  measures "d509" distance of L1.end L2.end
  measures "d510" distance of L0.end L1.end
  measures "d512" distance between parallel lines of L8 L3
  measures "d513" diameter of A0
  measures "d514" diameter of A1
  measures "d515" diameter of A2
  measures "d516" diameter of A3
  measures "d527" diameter of A4
  measures "d532" diameter of A5
sketch "Skizze88" plane through (102.8, 0.0934, -17.5) normal (-1, 0, 0) x (0, 0, 1)
  circle A0 centre (0, 0) radius 12 projected
  circle A1 centre (0, 0) radius 14
  circle A2 centre (0, 0) radius 12
  point P0 (17.5, -0.0934)
  dimension "d773" = 2
  constraints: 2 centre point, 2 coincident, 1 concentric
  measures "d773" radial gap between concentric circles of A0 A1
extrude "Extrusion77" add sketch "Skizze88" against normal blind 6 bodies 1
sketch "Skizze81" plane through (104.3, 0.0934, -17.5) normal (1, 0, 0) x (0, -1, 0)
  circle A0 centre (0, 0) radius 10.5 projected
  circle A1 centre (0, 0) radius 10.5
  point P0 (-6.0612, 8.5739)
  point P1 (-6.0612, -8.5739)
  point P2 (0.0934, -17.5)
  constraints: 1 centre point, 1 coincident
extrude "Extrusion69" add sketch "Skizze81" along normal blind 2 bodies 1
extrude "Extrusion70" [suppressed]
extrude "Extrusion110" [suppressed]
sketch "Skizze76" plane through (104.3, 0.0934, -17.5) normal (1, 0, 0) x (0, 0, -1)
  circle A0 centre (0, 0) radius 10.5 projected
  circle A1 centre (0, 0) radius 6
  point P0 (-17.5, -0.0934)
  dimension "d506" = 12
  constraints: 1 centre point, 1 coincident
  measures "d506" diameter of A1
extrude "Extrusion60" [suppressed]
sketch "Skizze82" plane through (106.3, 0.0934, -17.5) normal (1, 0, 0) x (0, 0, -1)
  circle A0 centre (0, 0) radius 6 projected
  circle A1 centre (0, 0) radius 10.5 projected
  circle A2 centre (0, 0) radius 6
  point P0 (-17.5, -0.0934)
  constraints: 1 centre point, 1 coincident, 1 concentric
ref_plane "Arbeitsebene41" through (104.55, 0.0934, -17.5) normal (1, 0, 0) x (0, 0, -1)
sketch "Skizze116" plane through (104.55, 0.0934, -17.5) normal (1, 0, 0) x (0, 0, -1)
  point P0 (-17.5, -0.0934)
sketch "Skizze115" plane through (106.3, 0.0934, -17.5) normal (1, 0, 0) x (0, 0, -1)
  circle A0 centre (0, 0) radius 10.5 projected
  circle A1 centre (0, 0) radius 11.25
  point P0 (-17.5, -0.0934)
  dimension "d672" = 22.5
  constraints: 1 centre point, 1 coincident
  measures "d672" diameter of A1
extrude "Extrusion87" cut sketch "Skizze115" along normal blind 2.2 contours A0 | A1 bodies 1
sketch "Skizze134" plane through (102.8, 0.0934, -17.5) normal (-1, 0, 0) x (0, 0, 1)
  line L0 (-7, -10.4434) -> (5.6, -10.4434)
  line L1 (8.3, -7.7434) -> (8.3, 7.5566)
  line L2 (5.6, 10.2566) -> (-7, 10.2566)
  line L3 (-9.7, 7.5566) -> (-9.7, -7.7434)
  line L4 (-9.7, -10.4434) -> (8.3, 10.2566) construction
  line L5 (8.3, -10.4434) -> (-9.7, 10.2566) construction
  arc A0 (8.3, 7.5566) -> (5.6, 10.2566) centre (5.6, 7.5566) ccw
  arc A1 (5.6, -10.4434) -> (8.3, -7.7434) centre (5.6, -7.7434) ccw
  arc A2 (-9.7, -7.7434) -> (-7, -10.4434) centre (-7, -7.7434) ccw
  arc A3 (-7, 10.2566) -> (-9.7, 7.5566) centre (-7, 7.5566) ccw
  circle A4 centre (5, 7.6566) radius 1.05 projected
  point P0 (17.5, -0.0934)
  point P1 (-0.7, -0.0934)
  dimension "d730" = 18
  dimension "d731" = 20.7
  dimension "d732" = 2.7
  dimension "d733" = 14.7
  constraints: 12 end point, 8 point on circle, 8 point on line, 8 tangent, 4 centre point, 3 equal radius, 2 midpoint, 2 parallel, 1 horizontal, 1 perpendicular
  measures "d730" distance of L5.end L4.end
  measures "d731" distance of L4.end L5.start
  measures "d732" radius of A0
  measures "d733" distance from line of A4.centre L3
split body "Trennen10" result two bodies by plane through (0, 0, -17.6) normal (0, 0, -1) bodies 1 first body at (61.9493, 2.4733, -35.6271)
sketch "Skizze83" plane through (73.9362, 3.7, -25.1) normal (0, 0, -1) x (-1, 0, 0)
  circle A0 centre (2.1362, -3.7) radius 2.55 projected
  line L0 (6.4086, -3.7) -> (4.2724, 0) projected
  line L1 (4.2724, 0) -> (0, 0) projected
  line L2 (0, 0) -> (-2.1362, -3.7) projected
  line L3 (-2.1362, -3.7) -> (0, -7.4) projected
  line L4 (0, -7.4) -> (4.2724, -7.4) projected
  line L5 (4.2724, -7.4) -> (6.4086, -3.7) projected
  point P0 (73.9362, -3.7)
extrude "Innenbolzenverstärkung1" [suppressed]
sketch "Skizze84" plane through (69.6638, -3.7, -10.1) normal (0, 0, 1) x (1, 0, 0)
  circle A0 centre (2.1362, 3.7) radius 2.55 projected
  line L0 (0, 7.4) -> (-2.1362, 3.7) projected
  line L1 (-2.1362, 3.7) -> (0, 0) projected
  line L2 (0, 0) -> (4.2724, 0) projected
  line L3 (4.2724, 0) -> (6.4086, 3.7) projected
  line L4 (6.4086, 3.7) -> (4.2724, 7.4) projected
  line L5 (4.2724, 7.4) -> (0, 7.4) projected
  point P0 (-69.6638, 3.7)
extrude "Innenbolzenverstärkung2" [suppressed]
ref_plane "Arbeitsebene38" through (124.8, 0, -17.5) normal (1, 0, 0) x (0, 0, -1)
sketch "Skizze100" plane through (124.8, 0, -17.5) normal (1, 0, 0) x (0, 0, -1)
  circle A0 centre (0, 0) radius 12.5
  point P0 (-17.5, 0)
  dimension "d588" = 25
  constraints: 1 centre point
  measures "d588" diameter of A0
sketch "Skizze117" plane through (106.3, 0.0934, -17.5) normal (1, 0, 0) x (0, 0, -1)
  circle A0 centre (0, 0) radius 6 projected
  circle A1 centre (0, 0) radius 10.85
  point P0 (-17.5, -0.0934)
  dimension "d675" = 21.7
  constraints: 1 centre point, 1 coincident
  measures "d675" diameter of A1
extrude "DämpferInnenscheibe" add sketch "Skizze117" along normal blind 2 separate body contours A0 | A1
sketch "Skizze118" plane through (106.3, 0.0934, -17.5) normal (-1, 0, 0) x (0, 0, 1)
  circle A0 centre (0, 0) radius 10.85 projected
  circle A1 centre (0, 0) radius 6
  circle A2 centre (0, 0) radius 7
  point P0 (17.5, -0.0934)
  dimension "d678" = 12
  dimension "d683" = 1
  constraints: 2 centre point, 2 coincident
  measures "d678" diameter of A1
  measures "d683" radial gap between concentric circles of A2 A1
ref_plane "Arbeitsebene55" through (113.3, 0.0934, -17.5) normal (1, 0, 0) x (0, 0, -1)
sketch "Skizze119" plane through (113.3, 0.0934, -17.5) normal (1, 0, 0) x (0, 0, -1)
  line L0 (0.1, 2.1066) -> (0.1, -0.0934) projected
  circle A0 centre (0.1, -0.0934) radius 10
  point P0 (-17.5, -0.0934)
  dimension "d774" = 20
  constraints: 1 centre point, 1 coincident
  measures "d774" diameter of A0
feature "Erhebung13" [suppressed]
sketch "Skizze140" plane through (113.3, 0, -17.6) normal (1, 0, 0) x (0, 0, -1)
  circle A0 centre (0, 0) radius 12.25
  point P0 (-17.6, 0)
  dimension "d777" = 24.5
  constraints: 1 centre point
  measures "d777" diameter of A0
extrude "Extrusion100" [suppressed]
fillet "Rundung37" [suppressed]
feature "Erhebung14" [suppressed]
fillet "Rundung36" [suppressed]
feature "Forminnen" [suppressed]
sketch "Skizze120" plane through (106.3, 0.0934, -17.5) normal (-1, 0, 0) x (0, 0, 1)
  circle A0 centre (0, 0) radius 10.85 projected
  circle A1 centre (0, 0) radius 15
  point P0 (17.5, -0.0934)
  dimension "d696" = 30
  constraints: 1 centre point, 1 coincident
  measures "d696" diameter of A1
extrude "Extrusion89" [suppressed]
sketch "Skizze139" plane through (109.8, 0.0934, -17.5) normal (1, 0, 0) x (0, 0, -1)
  line L0 (0.1, 2.1066) -> (0.1, -0.0934) projected
  circle A0 centre (0.1, -0.0934) radius 15
  point P0 (-17.5, -0.0934)
  constraints: 1 centre point
extrude "Extrusion98" [suppressed]
fillet "Rundung33" [suppressed]
sketch "Skizze122" plane through (106.3, 0.0934, -17.5) normal (-1, 0, 0) x (0, 0, 1)
  circle A0 centre (0, 0) radius 15 projected
  circle A1 centre (0, 0) radius 11.05
  point P0 (17.5, -0.0934)
  dimension "d700" = 22.1
  constraints: 1 centre point, 1 coincident
  measures "d700" diameter of A1
extrude "Extrusion90" [suppressed]
sketch "Skizze124" plane through (109.8, 0.0934, -17.5) normal (-1, 0, 0) x (0, 0, 1)
  line L0 (-13, 0) -> (13, 0)
  line L1 (0, 14) -> (0, 24) construction
  circle A0 centre (0, 0) radius 14
  point P0 (17.5, -0.0934)
  constraints: 2 end point, 1 vertical alignment, 2 other
extrude "Extrusion99" [suppressed]
fillet "Rundung34" [suppressed]
ref_plane "Arbeitsebene67" through (115.8, 0.0934, -17.5) normal (-1, 0, 0) x (0, 0, 1)
feature "Kombinieren10" [suppressed]
sketch "Skizze125" plane through (115.8, 0.0934, -17.5) normal (-1, 0, 0) x (0, 0, 1)
  circle A0 centre (0, 0) radius 18.8652
  point P0 (17.5, -0.0934)
  constraints: 1 centre point